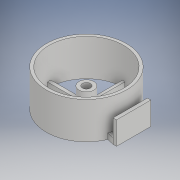
# Autodesk Inventor part: BasicThrustMotorHousing
Saved by Autodesk Inventor 2019 (Build 230136000, 136)
## iProperties
Created: 2018-09-19
Part Number: BasicThrustMotorHousing
Material: Generic
Document SubType Name: Modeling
Designer: hale985
Density: 1 g/cm^3
Appearance: Default
Author: hale985
Autodesk Inventor part; units mm, degrees
ref_plane "YZ Plane" through (0, 0, 0) normal (1, 0, 0) x (0, 1, 0)
ref_plane "XZ Plane" through (0, 0, 0) normal (0, 1, 0) x (-1, 0, 0)
ref_plane "XY Plane" through (0, 0, 0) normal (0, 0, 1) x (1, 0, 0)
sketch "Sketch1" plane through (0, 0, 0) normal (1, 0, 0) x (0, 1, 0)
  circle A0 centre (0, 0) radius 4.445
  circle A1 centre (0, 0) radius 8.255
  dimension "d0" = 8.89
  dimension "d1" = 3.81
  constraints: 2 centre point, 1 coincident
  measures "d0" diameter of A0
  measures "d1" radial gap between concentric circles of A0 A1
extrude "Extrusion1" add sketch "Sketch1" along normal blind 19.812
sketch "Sketch2" plane through (0, 0, 0) normal (-1, 0, 0) x (0, 0, 1)
  circle A0 centre (0, 0) radius 8.255
  circle A1 centre (0, 0) radius 7.747
  circle A2 centre (0, 0) radius 8.255 projected
  dimension "d42" = 0
  constraints: 2 centre point, 2 coincident
  measures "d42" radial gap between concentric circles of A2 A0
extrude "Extrusion2" add sketch "Sketch2" along normal blind 2.54 contours A0 | A1
sketch "Sketch3" plane through (-2.54, 0, 0) normal (-1, 0, 0) x (0, 0, 1)
  line L0 (19.05, 48.5955) -> (-19.05, 48.5955)
  circle A0 centre (0, 0) radius 8.255 projected
  line L1 (8.255, 0) -> (19.05, 48.5955)
  line L2 (-8.255, 0) -> (-19.05, 48.5955)
  arc A1 (8.255, 0) -> (-8.255, 0) centre (0, 0) ccw
  line L3 (-14.3008, 44.7855) -> (14.3008, 44.7855)
  line L4 (14.3008, 44.7855) -> (6.5962, 10.1022)
  arc A2 (6.5962, 10.1022) -> (-6.5962, 10.1022) centre (0, 0) ccw
  line L5 (-6.5962, 10.1022) -> (-14.3008, 44.7855)
  dimension "d6" = 38.1
  dimension "d7" = 19.05
  dimension "d8" = 3.81
  constraints: 12 end point, 6 point on circle, 2 centre point, 1 concentric, 1 horizontal, 3 other
  measures "d6" distance of L0.start L0.end
  measures "d7" horizontal distance of L0.start point (0, 0)
  measures "d8" distance between parallel lines of L0 L3
extrude "Extrusion3" add sketch "Sketch3" against normal blind 6.35 contours L1 A0 L2 L0
sketch "Sketch6" plane through (-2.54, 44.7855, -14.3008) normal (0, -1, 0) x (1, 0, 0)
  line L0 (6.35, 32.4159) -> (26.9875, 32.4159) projected
  line L1 (13.4874, 32.4159) -> (13.4874, 26.0989)
  line L2 (26.9875, 32.4159) -> (26.9875, -3.9117) projected
  point P0 (2.54, 14.3008)
  dimension "d20" = 13.5001
  constraints: 2 end point, 1 point on line, 1 vertical
  measures "d20" distance between parallel lines of L2 L1
sketch "Sketch10" plane through (0, 0, 0) normal (1, 0, 0) x (0, 0, -1)
  circle A0 centre (0, 0) radius 1.4542
  line L0 (-4.445, 1.4542) -> (4.445, 1.4542)
  line L1 (4.445, 1.4542) -> (4.445, -1.4542)
  line L2 (4.445, -1.4542) -> (-4.445, -1.4542)
  line L3 (-4.445, -1.4542) -> (-4.445, 1.4542)
  circle A1 centre (0, 0) radius 4.445 projected
  dimension "d43" = 0
  dimension "d44" = 0
  constraints: 8 end point, 2 parallel, 1 centre point, 1 coincident, 1 horizontal, 1 perpendicular
  measures "d43" distance edge to line of A1 L1
  measures "d44" distance edge to line of A1 L3
extrude "Extrusion7" cut sketch "Sketch10" against normal blind 22.225 contours A0 | A0 L0 A1 L2 | A0 L2 A1 L0 | A1 L3 L0 | L0 L1 A1 | A1 L1 L2 | L2 L3 A1
sketch "Sketch13" plane through (-2.54, 48.5955, 19.05) normal (0, 1, 0) x (1, 0, 0)
  line L0 (4.6355, 36.83) -> (1.7145, 36.83)
  line L1 (1.7145, 36.83) -> (1.7145, 33.909)
  line L2 (1.7145, 33.909) -> (4.6355, 33.909)
  line L3 (4.6355, 33.909) -> (4.6355, 36.83)
  line L4 (6.35, 38.1) -> (6.35, 0) projected
  line L5 (0, 38.1) -> (6.35, 38.1) projected
  line L6 (4.6228, 4.191) -> (1.7018, 4.191)
  line L7 (1.7018, 4.191) -> (1.7018, 1.27)
  line L8 (1.7018, 1.27) -> (4.6228, 1.27)
  line L9 (4.6228, 1.27) -> (4.6228, 4.191)
  line L10 (0, 0) -> (6.35, 0) projected
  line L11 (0, 0) -> (0, 38.1) projected
  line L12 (0, 0) -> (6.35, 0) projected
  line L13 (6.35, 38.1) -> (6.35, 0) projected
  line L14 (0, 38.1) -> (6.35, 38.1) projected
  point P0 (2.54, 19.05)
  dimension "d32" = 2.921
  dimension "d33" = 2.921
  dimension "d34" = 1.7145
  dimension "d35" = 1.27
  dimension "d36" = 2.921
  dimension "d37" = 2.921
  dimension "d38" = 1.7272
  dimension "d39" = 1.27
  constraints: 16 end point, 4 parallel, 2 horizontal, 2 perpendicular
  measures "d32" distance of L1.end L2.end
  measures "d33" distance of L0.end L1.end
  measures "d34" distance between parallel lines of L4 L3
  measures "d35" distance between parallel lines of L5 L0
  measures "d36" distance of L8.end L7.end
  measures "d37" distance of L7.end L6.end
  measures "d38" distance between parallel lines of L4 L9
  measures "d39" distance between parallel lines of L10 L8
extrude "Extrusion9" add sketch "Sketch13" along normal blind 3.81 contours L3 L2 L1 L0 | L4 L10 L11 L5 | L9 L8 L7 L6
sketch "Sketch14" plane through (0, 0, 0) normal (-1, 0, 0) x (0, 0, 1)
  arc A0 (4.2004, -1.4542) -> (4.445, 0) centre (0, 0) ccw projected
  line L0 (4.2004, -1.4542) -> (4.445, -1.4542) projected
  line L1 (4.445, -1.4542) -> (4.445, 0) projected
  arc A1 (4.445, 0) -> (4.2004, 1.4542) centre (0, 0) ccw projected
  line L2 (4.445, 0) -> (4.445, 1.4542) projected
  line L3 (4.445, 1.4542) -> (4.2004, 1.4542) projected
  arc A2 (-4.445, 0) -> (-4.2004, -1.4542) centre (0, 0) ccw projected
  line L4 (-4.445, 0) -> (-4.445, -1.4542) projected
  line L5 (-4.445, -1.4542) -> (-4.2004, -1.4542) projected
  arc A3 (-4.2004, 1.4542) -> (-4.445, 0) centre (0, 0) ccw projected
  line L6 (-4.2004, 1.4542) -> (-4.445, 1.4542) projected
  line L7 (-4.445, 1.4542) -> (-4.445, 0) projected
extrude "Extrusion10" add sketch "Sketch14" along normal blind 2.54
sketch "Sketch15" plane through (-2.54, 0, 0) normal (-1, 0, 0) x (0, 0, 1)
  circle A0 centre (0, 0) radius 41.275
  circle A1 centre (0, 0) radius 44.45
  dimension "d47" = 82.55
  dimension "d48" = 88.9
  constraints: 2 centre point, 2 coincident
  measures "d47" diameter of A0
  measures "d48" diameter of A1
extrude "Extrusion11" add sketch "Sketch15" against normal blind 2.54
sketch "Sketch16" plane through (0, 0, 0) normal (1, 0, 0) x (0, 0, -1)
  circle A0 centre (0, 0) radius 44.45
  circle A1 centre (0, 0) radius 41.275
  dimension "d51" = 82.55
  constraints: 2 centre point, 2 coincident
  measures "d51" diameter of A1
extrude "Extrusion12" add sketch "Sketch16" along normal blind 38.1
sketch "Sketch19" plane through (-2.54, 0, 0) normal (-1, 0, 0) x (0, 0, 1)
  line L0 (4.2004, 1.4542) -> (-4.2004, 1.4542) projected
  arc A0 (-16.6452, 37.7699) -> (16.6452, 37.7699) centre (0, 0) ccw projected
  line L1 (-4.2004, 1.4542) -> (-41.2494, 1.4542)
  line L2 (4.2004, 1.4542) -> (41.2494, 1.4542)
  circle A1 centre (0, 0) radius 8.382
  line L3 (-4.2004, -1.4542) -> (4.2004, -1.4542)
  line L4 (4.2004, 1.4542) -> (-4.2004, 1.4542)
  line L5 (-41.2494, -1.4542) -> (41.2494, -1.4542)
  constraints: 10 end point, 4 point on circle, 2 horizontal, 1 centre point, 1 coincident, 1 parallel, 1 point on line
extrude "Extrusion14" add sketch "Sketch19" against normal blind 6.35 contours L2 A1 L5 L3 L1 L0 | L2 A0 L5 A1 | A1 L5 A0 L1
sketch "Sketch20" plane through (3.81, 0, 0) normal (1, 0, 0) x (0, 0, -1)
  arc A0 (4.2004, -1.4542) -> (4.2004, 1.4542) centre (0, 0) ccw projected
  line L0 (4.2004, 1.4542) -> (-4.2004, 1.4542) projected
  arc A1 (-4.2004, 1.4542) -> (-4.2004, -1.4542) centre (0, 0) ccw projected
  line L1 (-4.2004, -1.4542) -> (4.2004, -1.4542) projected
extrude "Extrusion15" cut sketch "Sketch20" against normal blind 6.35
sketch "Sketch21" plane through (-2.54, 0, 0) normal (-1, 0, 0) x (0, 0, 1)
  arc A0 (-8.1259, -1.4542) -> (8.1259, -1.4542) centre (0, 0) ccw projected
  line L0 (1.8212, -8.0516) -> (1.8212, -41.2348)
  arc A1 (-41.2494, -1.4542) -> (41.2494, -1.4542) centre (0, 0) ccw projected
  line L1 (-1.8492, -41.2336) -> (-1.8492, -8.1755)
  arc A2 (-1.8492, -41.2336) -> (1.8212, -41.2348) centre (0, 0) ccw
  line L2 (-1.8492, -8.1755) -> (-1.8492, -8.0452)
  constraints: 6 end point, 6 point on circle, 3 vertical, 1 centre point
extrude "Extrusion16" add sketch "Sketch21" against normal blind 6.35
sketch "Sketch23" plane through (3.81, 0, 0) normal (1, 0, 0) x (0, 0, -1)
  line L0 (19.05, 52.4055) -> (-19.05, 52.4055) projected
  line L1 (-19.05, 48.5955) -> (-19.05, 52.4055) projected
  line L2 (19.05, 52.4055) -> (-19.05, 52.4055)
  line L3 (-19.05, 52.4055) -> (-19.05, 48.5955)
  line L4 (-19.05, 48.5955) -> (19.05, 48.5955)
  line L5 (19.05, 48.5955) -> (19.05, 52.4055)
  point P0 (0, 0)
  constraints: 8 end point, 2 parallel, 1 horizontal, 1 perpendicular
extrude "Extrusion17" add sketch "Sketch23" along normal blind 19.05
body "Solid1"
